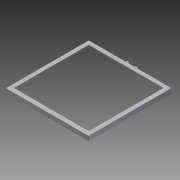
# Autodesk Inventor part: Propane Burner Lid
Saved by Autodesk Inventor 2013 SP2 (Build 170200200, 200)
## iProperties
Created: 2014-05-30
Part Number: Propane Burner Lid
Material: Steel
Document SubType Name: Modeling
Designer: jmw3
Mass: 1138.65 g
Surface Area: 1904.45 cm^2
Volume: 145.051 cm^3
Density: 7.85 g/cm^3
Author: jmw3
Autodesk Inventor part; units mm, degrees
ref_plane "YZ Plane" through (0, 0, 0) normal (1, 0, 0) x (0, 1, 0)
ref_plane "XZ Plane" through (0, 0, 0) normal (0, 1, 0) x (-1, 0, 0)
ref_plane "XY Plane" through (0, 0, 0) normal (0, 0, 1) x (1, 0, 0)
sketch "Sketch1" plane through (0, 0, 0) normal (0, 1, 0) x (-1, 0, 0)
  line L0 (-330.1619, 330.1619) -> (330.1619, 330.1619)
  line L1 (330.1619, 330.1619) -> (330.1619, -330.1619)
  line L2 (330.1619, -330.1619) -> (-330.1619, -330.1619)
  line L3 (-330.1619, -330.1619) -> (-330.1619, 330.1619)
  line L4 (0, -464.4492) -> (0, 464.4492) projected
  line L5 (464.4492, 0) -> (-464.4492, 0) projected
  line L6 (0, -464.4492) -> (0, 464.4492) projected
  line L7 (-331.7494, 331.7494) -> (331.7494, 331.7494)
  line L8 (331.7494, 331.7494) -> (331.7494, -331.7494)
  line L9 (331.7494, -331.7494) -> (-331.7494, -331.7494)
  line L10 (-331.7494, -331.7494) -> (-331.7494, 331.7494)
  point P0 (0, 0)
  dimension "d0" = 660.3238
  dimension "d2" = 660.3238
  dimension "d3" = 1.5875
  dimension "d4" = 1.5875
  constraints: 16 end point, 4 parallel, 2 horizontal, 2 perpendicular, 4 other
  measures "d0" distance between parallel lines of L1 L3
  measures "d2" distance between parallel lines of L2 L0
  measures "d3" distance between parallel lines of L10 L3
  measures "d4" distance between parallel lines of L0 L7
extrude "Extrusion1" add sketch "Sketch1" against normal blind 36.5125 contours L3 L5 L10 L7 L4 L0 | L4 L7 L8 L5 L1 L0 | L3 L2 L4 L9 L10 L5 | L5 L8 L9 L4 L2 L1
sketch "Sketch2" plane through (0, 0, 0) normal (0, 1, 0) x (1, 0, 0)
  line L0 (331.7494, -331.7494) -> (-331.7494, -331.7494) projected
  line L1 (331.7494, 331.7494) -> (331.7494, -331.7494) projected
  line L2 (-331.7494, -331.7494) -> (331.7494, -331.7494)
  line L3 (331.7494, -331.7494) -> (331.7494, 331.7494)
  line L4 (331.7494, 331.7494) -> (-331.7494, 331.7494)
  line L5 (-331.7494, 331.7494) -> (-331.7494, -331.7494)
  line L6 (-299.9994, 299.9994) -> (299.9994, 299.9994)
  line L7 (299.9994, 299.9994) -> (299.9994, -299.9994)
  line L8 (299.9994, -299.9994) -> (-299.9994, -299.9994)
  line L9 (-299.9994, -299.9994) -> (-299.9994, 299.9994)
  line L10 (0, 464.4492) -> (0, -464.4492) projected
  line L11 (-464.4492, 0) -> (464.4492, 0) projected
  line L12 (-331.7494, 331.7494) -> (331.7494, 331.7494) projected
  line L13 (-331.7494, -331.7494) -> (-331.7494, 331.7494) projected
  point P0 (0, 0)
  dimension "d146" = 31.75
  dimension "d147" = 31.75
  constraints: 16 end point, 4 parallel, 2 horizontal, 2 perpendicular, 2 other
  measures "d146" distance between parallel lines of L12 L6
  measures "d147" distance between parallel lines of L13 L9
extrude "Extrusion2" add sketch "Sketch2" along normal blind 1.5875 contours L0 L10 L8 L7 L11 L1 | L0 L5 L11 L9 L8 L10 | L11 L7 L6 L10 L4 L1 | L5 L4 L10 L6 L9 L11
fillet "Fillet1" radius 3.175 8 edges at (0, 1.5875, 331.7494) (331.7494, -17.4625, 331.7494) (331.7494, 1.5875, 0) (-331.7494, -17.4625, 331.7494) (-331.7494, 1.5875, 0) (0, 1.5875, -331.7494) (331.7494, -17.4625, -331.7494) (-331.7494, -17.4625, -331.7494)
sketch "Sketch3" plane through (328.5744, -36.5125, -331.7494) normal (0, 0, -1) x (-1, 0, 0)
  line L0 (657.1488, 38.1) -> (0, 38.1) projected
  line L1 (-3.175, 34.925) -> (-3.175, 0) projected
  line L2 (660.3238, 0) -> (660.3238, 34.925) projected
  line L3 (328.5744, -7.62) -> (328.5744, 45.72) projected
  line L4 (284.1244, 28.575) -> (303.1744, 28.575)
  line L5 (303.1744, 28.575) -> (303.1744, 9.525)
  line L6 (303.1744, 9.525) -> (284.1244, 9.525)
  line L7 (284.1244, 9.525) -> (284.1244, 28.575)
  point P0 (328.5744, 36.5125)
  dimension "d12" = 19.05
  dimension "d14" = 9.525
  dimension "d15" = 19.05
  dimension "d145" = 25.4
  constraints: 8 end point, 2 parallel, 1 horizontal, 1 perpendicular
  measures "d12" distance between parallel lines of L6 L4
  measures "d14" distance between parallel lines of L0 L4
  measures "d15" distance between parallel lines of L5 L7
  measures "d145" distance between parallel lines of L3 L5
extrude "Extrusion3" add sketch "Sketch3" along normal blind 19.05
sketch "Sketch4" plane through (25.4, -7.9375, -331.7494) normal (0, 1, 0) x (1, 0, 0)
  line L0 (0, 19.05) -> (19.05, 19.05) projected
  line L1 (0, 0) -> (0, 19.05) projected
  circle A0 centre (9.525, 9.525) radius 3.175
  point P0 (-25.4, -331.7494)
  dimension "d19" = 6.35
  dimension "d21" = 9.525
  dimension "d22" = 9.525
  constraints: 1 centre point
  measures "d19" diameter of A0
  measures "d21" distance from line of L1 A0.centre
  measures "d22" distance from line of L0 A0.centre
extrude "Extrusion4" cut sketch "Sketch4" against normal up to next
fillet "Fillet2" radius 1.5875 7 edges at (44.45, -26.9875, -341.2744) (44.45, -17.4625, -350.7994) (44.45, -7.9375, -341.2744) (34.925, -7.9375, -350.7994) (34.925, -26.9875, -350.7994) (25.4, -17.4625, -350.7994) (25.4, -7.9375, -341.2744)
fillet "Fillet3" radius 1.5875 2 edges at (25.865, -26.5225, -350.3344) (25.4, -26.9875, -340.4806)
mirror "Mirror1" about plane through (0, 0, 0) normal (1, 0, 0) of "Extrusion3", "Fillet2", "Extrusion4"
sketch "Sketch5" plane through (328.5744, -36.5125, -350.7994) normal (0, 0, -1) x (-1, 0, 0)
  line L0 (285.7119, 26.9875) -> (301.5869, 26.9875) projected
  line L1 (285.7119, 11.1125) -> (285.7119, 26.9875) projected
  circle A0 centre (293.6494, 19.05) radius 3.175
  point P0 (328.5744, 36.5125)
  dimension "d27" = 6.35
  dimension "d28" = 7.9375
  dimension "d29" = 7.9375
  constraints: 1 centre point
  measures "d27" diameter of A0
  measures "d28" distance from line of L1 A0.centre
  measures "d29" distance from line of L0 A0.centre
sketch "Sketch6" plane through (331.7494, -36.5125, -328.5744) normal (1, 0, 0) x (0, 0, -1)
  line L0 (-328.5744, -7.62) -> (-328.5744, 45.72) projected
  circle A0 centre (-57.15, 14.2875) radius 3.175
  line L1 (3.175, 0) -> (3.175, 34.925) projected
  circle A1 centre (-599.9988, 14.2875) radius 3.175
  line L2 (1.5875, 36.5125) -> (-658.7363, 36.5125) projected
  line L3 (-658.7363, 36.5125) -> (-658.7363, 0) projected
  point P0 (-328.5744, 36.5125)
  dimension "d36" = 6.35
  dimension "d37" = 60.325
  dimension "d142" = -58.7375
  constraints: 2 centre point, 1 symmetric about line, 1 other
  measures "d36" diameter of A0
  measures "d37" distance from line of L1 A0.centre
  measures "d142" distance from line of L3 A1.centre
body "Solid1"
